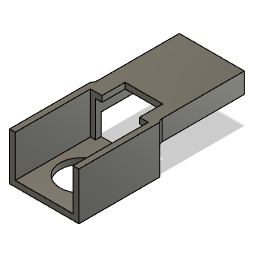
CMCz v3 (Autodesk Fusion 360 archive; units mm, degrees)
design "wire holder PIP modif"
Autodesk Fusion 360 part; units mm, degrees
note: some values were not read from the file. Chosen so that the rebuilt part matches the saved one: which face or edge a step refers to. Set by a fixed rule: which sketch regions a step uses.
sketch "Esquisse1" plane through (0, 0, 0) normal (0, 1, 0) x (1, 0, 0)
  line L0 (4.125, 6.5) -> (-4.125, 6.5)
  line L1 (-4.125, 6.5) -> (-4.125, -6.5)
  line L2 (-4.125, -6.5) -> (4.125, -6.5)
  line L3 (4.125, -6.5) -> (4.125, 6.5)
  line L4 (4.125, 6.5) -> (-4.125, -6.5) construction
  line L5 (-4.125, 6.5) -> (4.125, -6.5) construction
  line L6 (-5.625, -8) -> (5.625, -8)
  line L7 (5.625, -8) -> (5.625, 8)
  line L8 (5.625, 8) -> (-5.625, 8)
  line L9 (-5.625, 8) -> (-5.625, -8)
  line L10 (-1.375, 6.5) -> (-1.375, 8) construction
  line L11 (1.375, 6.5) -> (1.375, 8) construction
  line L12 (-1.875, 8) -> (-1.875, 6.5)
  line L13 (-0.875, 8) -> (-0.875, 6.5)
  line L14 (0.875, 8) -> (0.875, 6.5)
  line L15 (1.875, 8) -> (1.875, 6.5)
  line L16 (3.625, 8) -> (3.625, 6.5)
  line L17 (-3.625, 8) -> (-3.625, 6.5)
  line L18 (-4.125, -6.5) -> (-4.125, -8)
  line L19 (4.125, -6.5) -> (4.125, -4.6231)
  line L20 (4.125, -4.6231) -> (4.125, -8)
  dimension "d1" = 13
  dimension "d2" = 8.25
  dimension "d3" = 1.5
  dimension "d4" = 2.75
  dimension "d5" = 2.75
  dimension "d6" = 0.5
  dimension "d7" = 0.5
  dimension "d8" = 0.5
  dimension "d9" = 0.5
  dimension "d10" = 0.5
  dimension "d11" = 0.5
  dimension "d91" = 1.5
  constraint horizontal L0
  constraint perpendicular L0 L1
  constraint parallel L0 L2
  constraint parallel L1 L3
  constraint coincident L4 origin
  constraint coincident L5 origin
  constraint coincident L0 L10.start
  constraint coincident L8 L10.end
  constraint perpendicular L8 L10
  constraint coincident L0 L11.start
  constraint coincident L8 L11.end
  constraint perpendicular L8 L11
  constraint coincident L8 L12.start
  constraint coincident L0 L12.end
  constraint perpendicular L0 L12
  constraint coincident L8 L13.start
  constraint coincident L0 L13.end
  constraint perpendicular L0 L13
  constraint coincident L8 L14.start
  constraint coincident L0 L14.end
  constraint perpendicular L0 L14
  constraint coincident L8 L15.start
  constraint coincident L0 L15.end
  constraint perpendicular L0 L15
  constraint coincident L8 L16.start
  constraint coincident L0 L16.end
  constraint perpendicular L0 L16
  constraint coincident L8 L17.start
  constraint coincident L0 L17.end
  constraint perpendicular L0 L17
  constraint coincident L6 L18.end
  constraint perpendicular L6 L18
  constraint perpendicular L2 L19
  constraint coincident L6 L20.end
  constraint perpendicular L6 L20
  measures "d1" distance of L0.start L2.end
  measures "d2" distance of L0.start L0.end
  measures "d4" distance of L0.end L10.start
  measures "d5" distance of L10 L11
  measures "d6" horizontal distance of L0.end L17.start
  measures "d7" distance of L10 L12
  measures "d8" distance of L10 L13
  measures "d9" distance of L11 L14
  measures "d10" distance of L11 L15
  measures "d11" distance of L0.start L16
  measures "d91" distance of L1.end L18.end
extrude "Extrusion1" add sketch "Esquisse1" along normal blind 1
extrude "Extrusion2" add sketch "Esquisse1" against normal blind 2.5 contours L0 L3 L6 L7 L8 L16 L19 L20 | L0 L8 L14 L15 | L0 L1 L6 L8 L9 L17 L18 | L0 L8 L12 L13
sketch "Esquisse5" plane through (0, 1, 0) normal (0, 1, 0) x (-1, 0, 0)
  line L0 (5.625, -8) -> (5.625, 8)
  line L1 (5.625, 8) -> (-5.625, 8)
  line L2 (-5.625, 8) -> (-5.625, -8)
  line L3 (-5.625, -8) -> (5.625, -8)
  line L4 (5.625, 8) -> (-5.625, 8)
  line L5 (5, 8) -> (-5, 8)
  line L6 (-5, 8) -> (-5, 20)
  line L7 (-5, 20) -> (5, 20)
  line L8 (5, 20) -> (5, 8)
  line L9 (5.625, 8) -> (5.625, -8)
  line L10 (-5.625, -8) -> (-5.625, 8)
  line L11 (-6, 7) -> (-6, 21)
  line L12 (-6, 21) -> (6, 21)
  line L13 (6, 21) -> (6, 7)
  line L14 (6, 7) -> (-6, 7)
  line L15 (4.125, -6.5) -> (4.125, 8)
  line L16 (-4.125, 8) -> (-4.125, -6.5)
  point P0 (-4.125, 8)
  point P1 (0, 8)
  point P2 (0, 8)
  dimension "d33" = 10
  dimension "d34" = 12
  dimension "d35" = -1
  constraint horizontal L5
  constraint vertical L6
  constraint horizontal L7
  constraint vertical L8
  constraint coincident L5 P0
  constraint midpoint L4 P2
  constraint midpoint L5 P2
  constraint coincident P2 P1
  measures "d33" distance of L5.start L5.end
  measures "d34" distance of L5.end L6.end
extrude "Extrusion6" add sketch "Esquisse5" against normal blind 7.2 contours L0 L1 L4 L5 L9 L14 L15 | L0 L1 L2 L4 L6 L7 L8 L9 L10 L11 L12 L13 L14 | L1 L2 L4 L5 L10 L14 L16
sketch "Esquisse6" plane through (0, -6.2, 0) normal (0, -1, 0) x (1, 0, 0)
  line L0 (5, 20) -> (5, 8)
  line L1 (5, 8) -> (4.125, 8)
  line L2 (4.125, 8) -> (4.125, 7)
  line L3 (4.125, 7) -> (6, 7)
  line L4 (6, 7) -> (6, 21)
  line L5 (6, 21) -> (-6, 21)
  line L6 (-6, 21) -> (-6, 7)
  line L7 (-6, 7) -> (-4.125, 7)
  line L8 (-4.125, 7) -> (-4.125, 8)
  line L9 (-4.125, 8) -> (-5, 8)
  line L10 (-5, 8) -> (-5, 20)
  line L11 (-5, 20) -> (5, 20)
  line L12 (-6, 21) -> (6, 21)
  line L13 (6, 21) -> (6, 7)
  line L14 (6, 7) -> (-6, 7)
  line L15 (-6, 7) -> (-6, 21)
  circle A0 centre (0, 14.5) radius 3.75
  line L16 (0, 7) -> (0, 21) construction
  line L17 (-4.125, 8) -> (4.125, 8)
  dimension "d39" = 6.5
  dimension "d40" = 7.5
  constraint horizontal L12
  constraint vertical L13
  constraint horizontal L14
  constraint vertical L15
  constraint coincident L3.end L4.start
  constraint coincident L5.end L6.start
  constraint midpoint L14 L16.start
  constraint midpoint L5 L16.end
  constraint coincident A0.centre L16
  measures "d39" distance of A0.centre L17
  measures "d40" diameter of A0
extrude "Extrusion7" add sketch "Esquisse6" along normal blind 1
sketch "Esquisse9" plane through (0, 1, 0) normal (0, 1, 0) x (-1, 0, 0)
  line L0 (5, 8) -> (-5, 8)
  line L1 (-5, 8) -> (-5, 20)
  line L2 (-5, 20) -> (5, 20)
  line L3 (5, 20) -> (5, 8)
  line L4 (5.625, 7) -> (6, 7)
  line L5 (6, 7) -> (6, 21)
  line L6 (6, 21) -> (-6, 21)
  line L7 (-6, 21) -> (-6, 7)
  line L8 (-6, 7) -> (-5.625, 7)
  line L9 (-5.625, 7) -> (-5.625, -8)
  line L10 (-5.625, -8) -> (5.625, -8)
  line L11 (5.625, -8) -> (5.625, 7)
  line L12 (3, 8) -> (-3.5, 8)
  line L13 (-3.5, 8) -> (-3.5, 4)
  line L14 (-3.5, 4) -> (3, 4)
  line L15 (3, 4) -> (3, 8)
  dimension "d63" = 4
  dimension "d64" = 6.5
  dimension "d65" = 1.5
  constraint horizontal L12
  constraint vertical L13
  constraint horizontal L14
  constraint vertical L15
  constraint coincident L0 L12.start
  measures "d63" distance of L12.end L13.end
  measures "d64" distance of L13.end L14.end
  measures "d65" distance of L1 L12.end
extrude "Extrusion10" cut sketch "Esquisse9" against normal blind 2 contours L0 L12 L13 L14 L15
sketch "Esquisse10" plane through (0, 0, 7) normal (0, 0, -1) x (-1, 0, 0)
  line L0 (5.625, 1) -> (5.625, -2.5)
  line L1 (5.625, -2.5) -> (4.125, -2.5)
  line L2 (4.125, -2.5) -> (4.125, -6.2)
  line L3 (4.125, -6.2) -> (-4.125, -6.2)
  line L4 (-4.125, -6.2) -> (-4.125, -2.5)
  line L5 (-4.125, -2.5) -> (-5.625, -2.5)
  line L6 (-5.625, -2.5) -> (-5.625, 1)
  line L7 (-5.625, 1) -> (-6, 1)
  line L8 (-6, 1) -> (-6, -7.2)
  line L9 (-6, -7.2) -> (6, -7.2)
  line L10 (6, -7.2) -> (6, 1)
  line L11 (6, 1) -> (5.625, 1)
  line L12 (-6, -7.2) -> (6, -7.2)
  line L13 (6, -7.2) -> (6, -6.2)
  line L14 (6, -6.2) -> (-6, -6.2)
  line L15 (-6, -6.2) -> (-6, -7.2)
  line L16 (-5.625, -6.2) -> (-5.625, -7.2)
  line L17 (5.625, -6.2) -> (5.625, -7.2)
  constraint horizontal L12
  constraint vertical L13
  constraint horizontal L14
  constraint vertical L15
  constraint coincident L10 L13.end
  constraint coincident L8.end L9.start
  constraint collinear L3 L14
  constraint coincident L14 L16.start
  constraint coincident L12 L16.end
  constraint perpendicular L12 L16
  constraint coincident L14 L17.start
  constraint coincident L12 L17.end
  constraint perpendicular L12 L17
  constraint collinear L6 L16
  constraint collinear L0 L17
sketch "Esquisse11" plane through (0, -7.2, 0) normal (0, -1, 0) x (1, 0, 0)
  circle A0 centre (0, 14.5) radius 3.75
  line L0 (6, 7) -> (6, 21)
  line L1 (6, 21) -> (-6, 21)
  line L2 (-6, 21) -> (-6, 7)
  circle A1 centre (0, 4.5) radius 2.5
  line L3 (-6, 7) -> (6, 7)
  dimension "d72" = 10
  dimension "d73" = 5
  measures "d72" distance of A0.centre A1.centre
  measures "d73" diameter of A1
sketch "Esquisse12" plane through (0, -6.2, 0) normal (0, 1, 0) x (-1, 0, 0)
  line L0 (4.125, 7) -> (4.125, 8)
  line L1 (4.125, 8) -> (5, 8)
  line L2 (5, 8) -> (5, 20)
  line L3 (5, 20) -> (-5, 20)
  line L4 (-5, 20) -> (-5, 8)
  line L5 (-5, 8) -> (-4.125, 8)
  line L6 (-4.125, 8) -> (-4.125, 7)
  line L7 (-4.125, 7) -> (4.125, 7)
  circle A0 centre (0, 14.5) radius 3.75
  line L8 (4.125, 2.1) -> (4.125, 6)
  arc A1 (0.025, -2) -> (4.125, 2.1) centre (0.025, 2.1) ccw
  line L9 (-0.025, -2) -> (0.025, -2)
  arc A2 (-4.125, 2.1) -> (-0.025, -2) centre (-0.025, 2.1) ccw
  line L10 (-4.125, 6) -> (-4.125, 2.1)
  line L11 (-3.125, 6) -> (-4.125, 6)
  line L12 (-3.125, 9) -> (-3.125, 6)
  line L13 (-4, 9) -> (-3.125, 9)
  line L14 (-4, 19) -> (-4, 9)
  line L15 (4, 19) -> (-4, 19)
  line L16 (4, 9) -> (4, 19)
  line L17 (3.125, 9) -> (4, 9)
  line L18 (3.125, 6) -> (3.125, 9)
  line L19 (4.125, 6) -> (3.125, 6)
  line L20 (4.125, 7) -> (4.125, 6)
  line L21 (-4.125, 7) -> (-4.125, 6)
  line L22 (5.125, 1.85) -> (-5.125, 1.85)
  constraint coincident L0.start L7.end
  constraint coincident L6.end L7.start
  constraint parallel L7 L11
  constraint parallel L6 L12
  constraint parallel L5 L13
  constraint parallel L4 L14
  constraint parallel L3 L15
  constraint parallel L2 L16
  constraint parallel L1 L17
  constraint parallel L0 L18
  constraint tangent L8 A1
  constraint tangent A1 L9
  constraint tangent L9 A2
  constraint tangent A2 L10
sketch "Esquisse13" plane through (0, -7.2, 0) normal (0, -1, 0) x (1, 0, 0)
  line L0 (6, 7) -> (6, 21)
  line L1 (6, 21) -> (-6, 21)
  line L2 (-6, 21) -> (-6, 7)
  circle A0 centre (0, 14.5) radius 3.75
  circle A1 centre (0, 4.25) radius 3.5
  line L3 (-6, 7) -> (6, 7)
  dimension "d84" = 7
  measures "d84" diameter of A1
extrude "Extrusion15" cut 1 faces at (1.6667, -1.4, 20) along direction (0, 0, 1) blind 6
fillet "Congé3" radius 1 2 edges at (-5.625, -0.75, 7) (5.625, -0.75, 7)

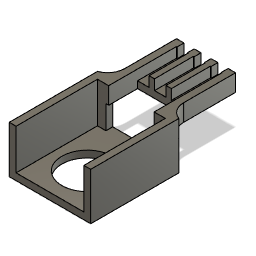
design "wire holder PIP midif v3"
Autodesk Fusion 360 part; units mm, degrees
sketch "Esquisse1" plane through (0, 0, 0) normal (0, 1, 0) x (1, 0, 0)
  line L0 (3.75, 4.5) -> (-3.75, 4.5)
  line L1 (-3.75, 4.5) -> (-3.75, -4.5)
  line L2 (-3.75, -4.5) -> (3.75, -4.5)
  line L3 (3.75, -4.5) -> (3.75, 4.5)
  line L4 (3.75, 4.5) -> (-3.75, -4.5) construction
  line L5 (-3.75, 4.5) -> (3.75, -4.5) construction
  line L6 (-4.75, -5.5) -> (4.75, -5.5)
  line L7 (4.75, -5.5) -> (4.75, 5.5)
  line L8 (4.75, 5.5) -> (-4.75, 5.5)
  line L9 (-4.75, 5.5) -> (-4.75, -5.5)
  line L10 (-1.25, 4.5) -> (-1.25, 5.5) construction
  line L11 (1.25, 4.5) -> (1.25, 5.5) construction
  line L12 (-1.75, 5.5) -> (-1.75, 4.5)
  line L13 (-0.75, 5.5) -> (-0.75, 4.5)
  line L14 (0.75, 5.5) -> (0.75, 4.5)
  line L15 (1.75, 5.5) -> (1.75, 4.5)
  line L16 (3.25, 5.5) -> (3.25, 4.5)
  line L17 (-3.25, 5.5) -> (-3.25, 4.5)
  line L18 (-3.75, -4.5) -> (-3.75, -5.5)
  line L19 (3.75, -4.5) -> (3.75, 15.3518)
  line L20 (3.75, 15.3518) -> (3.75, -5.5)
  line L21 (-1.65, 4.5) -> (-0.85, 4.5)
  line L22 (-0.85, 4.5) -> (-0.85, -5.5)
  line L23 (-0.85, -5.5) -> (-1.65, -5.5)
  line L24 (-1.65, -5.5) -> (-1.65, 4.5)
  line L25 (0.85, 4.5) -> (1.65, 4.5)
  line L26 (1.65, 4.5) -> (1.65, -5.5)
  line L27 (1.65, -5.5) -> (0.85, -5.5)
  line L28 (0.85, -5.5) -> (0.85, 4.5)
  line L29 (-3.35, 4.5) -> (-3.75, 4.5)
  line L30 (-3.75, 4.5) -> (-3.75, -5.5)
  line L31 (-3.75, -5.5) -> (-3.35, -5.5)
  line L32 (-3.35, -5.5) -> (-3.35, 4.5)
  line L33 (3.35, 4.5) -> (3.75, 4.5)
  line L34 (3.75, 4.5) -> (3.75, -5.5)
  line L35 (3.75, -5.5) -> (3.35, -5.5)
  line L36 (3.35, -5.5) -> (3.35, 4.5)
  line L37 (3.35, -5.5) -> (4.35, -5.5)
  line L38 (4.35, -5.5) -> (4.35, 5.5)
  line L39 (4.35, 5.5) -> (3.35, 5.5)
  line L40 (3.35, 5.5) -> (3.35, -5.5)
  line L41 (-3.35, -5.5) -> (-4.35, -5.5)
  line L42 (-4.35, -5.5) -> (-4.35, 5.5)
  line L43 (-4.35, 5.5) -> (-3.35, 5.5)
  line L44 (-3.35, 5.5) -> (-3.35, -5.5)
  dimension "d1" = 9
  dimension "d2" = 7.5
  dimension "d3" = 1
  dimension "d6" = 0.5
  dimension "d7" = 0.5
  dimension "d8" = 0.5
  dimension "d9" = 0.5
  dimension "d10" = 0.5
  dimension "d11" = 0.5
  dimension "d101" = 0.1
  dimension "d102" = 0.1
  dimension "d103" = 0.1
  dimension "d104" = 0.1
  dimension "d106" = 0.4
  dimension "d107" = 0.4
  dimension "d108" = 1.7
  dimension "d111" = 2.5
  dimension "d112" = 2.5
  dimension "d113" = 2.5
  dimension "d114" = 1.7
  dimension "d115" = 1.7
  dimension "d116" = 1
  dimension "d117" = 1
  constraint horizontal L0
  constraint perpendicular L0 L1
  constraint parallel L0 L2
  constraint parallel L1 L3
  constraint coincident L4 origin
  constraint coincident L5 origin
  constraint coincident L0 L10.start
  constraint coincident L8 L10.end
  constraint perpendicular L8 L10
  constraint coincident L0 L11.start
  constraint coincident L8 L11.end
  constraint perpendicular L8 L11
  constraint coincident L8 L12.start
  constraint coincident L0 L12.end
  constraint perpendicular L0 L12
  constraint coincident L8 L13.start
  constraint coincident L0 L13.end
  constraint perpendicular L0 L13
  constraint coincident L8 L14.start
  constraint coincident L0 L14.end
  constraint perpendicular L0 L14
  constraint coincident L8 L15.start
  constraint coincident L0 L15.end
  constraint perpendicular L0 L15
  constraint coincident L8 L16.start
  constraint coincident L0 L16.end
  constraint perpendicular L0 L16
  constraint coincident L8 L17.start
  constraint coincident L0 L17.end
  constraint perpendicular L0 L17
  constraint coincident L6 L18.end
  constraint perpendicular L6 L18
  constraint perpendicular L2 L19
  constraint coincident L6 L20.end
  constraint perpendicular L6 L20
  constraint horizontal L21
  constraint vertical L22
  constraint horizontal L23
  constraint vertical L24
  constraint coincident L0 L21.start
  constraint collinear L6 L23
  constraint horizontal L25
  constraint vertical L26
  constraint horizontal L27
  constraint vertical L28
  constraint coincident L6 L26.end
  constraint coincident L0 L25.start
  constraint horizontal L29
  constraint vertical L30
  constraint horizontal L31
  constraint vertical L32
  constraint coincident L0 L29.start
  constraint horizontal L33
  constraint vertical L34
  constraint horizontal L35
  constraint vertical L36
  constraint coincident L0 L33.start
  constraint horizontal L37
  constraint vertical L38
  constraint horizontal L39
  constraint vertical L40
  constraint coincident L8 L38.end
  constraint horizontal L41
  constraint vertical L42
  constraint horizontal L43
  constraint vertical L44
  constraint coincident L8 L42.end
  measures "d1" distance of L0.start L2.end
  measures "d2" distance of L0.start L0.end
  measures "d6" horizontal distance of L0.end L17.start
  measures "d7" distance of L10 L12
  measures "d8" distance of L10 L13
  measures "d9" distance of L11 L14
  measures "d10" distance of L11 L15
  measures "d11" distance of L0.start L16
  measures "d101" distance of L12 L24
  measures "d102" distance of L13 L22
  measures "d103" distance of L14 L28
  measures "d104" distance of L15 L26
  measures "d106" distance of L30 L32
  measures "d107" distance of L3 L36
  measures "d108" distance of L26 L36
  measures "d111" distance of L10 L30
  measures "d112" distance of L10 L11
  measures "d113" distance of L11 L34
  measures "d114" distance of L24 L32
  measures "d115" distance of L22 L28
  measures "d116" distance of L32 L42
  measures "d117" distance of L36 L38
extrude "Extrusion1" add sketch "Esquisse1" along normal blind 1 contours L0 L2 L3 L19 L20 L33 L34 L36 L40 | L3 L6 L8 L19 L20 L34 L37 L38 L39 | L0 L8 L19 L20 L33 L39 L40 | L0 L2 L26 L36 L40 | L0 L8 L16 L40 | L2 L6 L20 L34 L35 L36 L37 L40 | L0 L8 L15 L16 | L2 L6 L26 L36 L40 | L0 L8 L14 L15 L25 | L2 L6 L26 L27 L28 | L0 L2 L25 L26 L28 | L2 L6 L22 L28 | L0 L2 L22 L28 | L0 L8 L13 L14 | L2 L6 L22 L23 L24 | L0 L2 L21 L22 L24 | L0 L8 L12 L13 L21 | L2 L6 L24 L32 L44 | L0 L2 L24 L32 L44 | L0 L8 L12 L17 | L2 L6 L18 L30 L31 L32 L41 L44 | L0 L1 L2 L29 L30 L32 L44 | L0 L8 L17 L44 | L0 L1 L6 L8 L18 L29 L30 L41 L42 L43 L44
extrude "Extrusion2" add sketch "Esquisse1" against normal blind 1.75 contours L0 L2 L3 L19 L20 L33 L34 L36 L40 | L3 L6 L8 L19 L20 L34 L37 L38 L39 | L0 L8 L19 L20 L33 L39 L40 | L0 L8 L16 L40 | L2 L6 L20 L34 L35 L36 L37 L40 | L0 L8 L14 L15 L25 | L2 L6 L26 L27 L28 | L0 L2 L25 L26 L28 | L2 L6 L22 L23 L24 | L0 L2 L21 L22 L24 | L0 L8 L12 L13 L21 | L2 L6 L18 L30 L31 L32 L41 L44 | L0 L1 L2 L29 L30 L32 L44 | L0 L8 L17 L44 | L0 L1 L6 L8 L18 L29 L30 L41 L42 L43 L44
sketch "Esquisse5" plane through (0, 1, 0) normal (0, 1, 0) x (-1, 0, 0)
  line L0 (4.35, 5.5) -> (-4.35, 5.5)
  line L1 (-4.35, -5.5) -> (4.35, -5.5)
  line L2 (4.35, 5.5) -> (-4.35, 5.5)
  line L3 (5, 5.5) -> (-5, 5.5)
  line L4 (-5, 5.5) -> (-5, 17.5)
  line L5 (-5, 17.5) -> (5, 17.5)
  line L6 (5, 17.5) -> (5, 5.5)
  line L7 (4.75, 6.5) -> (4.75, -6.5)
  line L8 (-4.75, -6.5) -> (-4.75, 6.5)
  line L9 (-6, 4.5) -> (-6, 18.5)
  line L10 (-6, 18.5) -> (6, 18.5)
  line L11 (6, 18.5) -> (6, 4.5)
  line L12 (6, 4.5) -> (-6, 4.5)
  line L13 (3.75, -5.5) -> (3.75, 6.5)
  line L14 (-3.75, 6.5) -> (-3.75, -5.5)
  line L15 (-4.35, 5.5) -> (-4.35, -5.5)
  line L16 (4.35, -5.5) -> (4.35, 5.5)
  point P0 (0, 5.5)
  point P1 (0, 5.5)
  point P2 (-1.65, 5.5)
  point P3 (1.65, 5.5)
  point P4 (-3.35, 5.5)
  point P5 (-0.85, 5.5)
  point P6 (3.35, 5.5)
  point P7 (0.85, 5.5)
  dimension "d33" = 10
  dimension "d34" = 12
  dimension "d35" = -1
  constraint horizontal L3
  constraint vertical L4
  constraint horizontal L5
  constraint vertical L6
  constraint midpoint L2 P1
  constraint midpoint L3 P1
  constraint coincident P1 P0
  measures "d33" distance of L3.start L3.end
  measures "d34" distance of L3.end L4.end
extrude "Extrusion6" add sketch "Esquisse5" against normal blind 7.2 contours L0 L2 L3 L12 L13 L16 | L3 L7 L12 L16 | L3 L4 L5 L6 L7 L8 L9 L10 L11 L12 | L0 L2 L3 L12 L14 L15 | L3 L8 L12 L15
sketch "Esquisse6" plane through (0, -6.2, 0) normal (0, -1, 0) x (1, 0, 0)
  line L0 (5, 17.5) -> (5, 5.5)
  line L1 (5, 5.5) -> (3.75, 5.5)
  line L2 (3.75, 5.5) -> (3.75, 4.5)
  line L3 (3.75, 4.5) -> (6, 4.5)
  line L4 (6, 4.5) -> (6, 18.5)
  line L5 (6, 18.5) -> (-6, 18.5)
  line L6 (-6, 18.5) -> (-6, 4.5)
  line L7 (-6, 4.5) -> (-3.75, 4.5)
  line L8 (-3.75, 4.5) -> (-3.75, 5.5)
  line L9 (-3.75, 5.5) -> (-5, 5.5)
  line L10 (-5, 5.5) -> (-5, 17.5)
  line L11 (-5, 17.5) -> (5, 17.5)
  line L12 (-6, 18.5) -> (6, 18.5)
  line L13 (6, 18.5) -> (6, 4.5)
  line L14 (6, 4.5) -> (-6, 4.5)
  line L15 (-6, 4.5) -> (-6, 18.5)
  circle A0 centre (0, 12) radius 3.75
  line L16 (0, 4.5) -> (0, 18.5) construction
  line L17 (-3.35, 5.5) -> (-1.65, 5.5)
  line L18 (1.65, 5.5) -> (3.35, 5.5)
  line L19 (-0.85, 5.5) -> (0.85, 5.5)
  dimension "d40" = 7.5
  dimension "d133" = 6.5
  constraint horizontal L12
  constraint vertical L13
  constraint horizontal L14
  constraint vertical L15
  constraint coincident L3.end L4.start
  constraint coincident L5.end L6.start
  constraint midpoint L14 L16.start
  constraint midpoint L5 L16.end
  constraint coincident A0.centre L16
  measures "d40" diameter of A0
  measures "d133" distance of A0.centre L19
extrude "Extrusion7" add sketch "Esquisse6" along normal blind 1
sketch "Esquisse9" plane through (0, 1, 0) normal (0, 1, 0) x (-1, 0, 0)
  line L0 (-5, 5.5) -> (-5, 17.5)
  line L1 (-5, 17.5) -> (5, 17.5)
  line L2 (5, 17.5) -> (5, 5.5)
  line L3 (6, 4.5) -> (6, 18.5)
  line L4 (6, 18.5) -> (-6, 18.5)
  line L5 (-6, 18.5) -> (-6, 4.5)
  line L6 (-4.35, -5.5) -> (4.35, -5.5)
  line L7 (-4.35, 4.5) -> (-4.35, -5.5)
  line L8 (4.35, -5.5) -> (4.35, 4.5)
  line L9 (3.35, 5.5) -> (3.35, -4.5)
  line L10 (3.35, -4.5) -> (3.25, -4.5)
  line L11 (3.25, -4.5) -> (3.25, -5.5)
  line L12 (3.25, -5.5) -> (1.75, -5.5)
  line L13 (1.75, -5.5) -> (1.75, -4.5)
  line L14 (1.75, -4.5) -> (1.65, -4.5)
  line L15 (1.65, -4.5) -> (1.65, 5.5)
  line L16 (1.65, 5.5) -> (3.35, 5.5)
  line L17 (0.85, 5.5) -> (0.85, -4.5)
  line L18 (0.85, -4.5) -> (0.75, -4.5)
  line L19 (0.75, -4.5) -> (0.75, -5.5)
  line L20 (0.75, -5.5) -> (-0.75, -5.5)
  line L21 (-0.75, -5.5) -> (-0.75, -4.5)
  line L22 (-0.75, -4.5) -> (-0.85, -4.5)
  line L23 (-0.85, -4.5) -> (-0.85, 5.5)
  line L24 (-0.85, 5.5) -> (0.85, 5.5)
  line L25 (-3.25, -5.5) -> (-3.25, -4.5)
  line L26 (-3.25, -4.5) -> (-3.35, -4.5)
  line L27 (-3.35, -4.5) -> (-3.35, 5.5)
  line L28 (-3.35, 5.5) -> (-1.65, 5.5)
  line L29 (-1.65, 5.5) -> (-1.65, -4.5)
  line L30 (-1.65, -4.5) -> (-1.75, -4.5)
  line L31 (-1.75, -4.5) -> (-1.75, -5.5)
  line L32 (-1.75, -5.5) -> (-3.25, -5.5)
  line L33 (3.35, 5.5) -> (-3.35, 5.5)
  line L34 (-3.35, 5.5) -> (-3.35, 1.25)
  line L35 (-3.35, 1.25) -> (3.35, 1.25)
  line L36 (3.35, 1.25) -> (3.35, 5.5)
  dimension "d122" = 4.25
  constraint horizontal L33
  constraint vertical L34
  constraint horizontal L35
  constraint vertical L36
  constraint coincident L27 L34.end
  constraint coincident L9.start L16.end
  measures "d122" distance of L27.end L34.end
extrude "Extrusion10" cut sketch "Esquisse9" against normal blind 3.5 contours L27 L28 L29 L33 L34 L35 | L23 L29 L33 L35 | L17 L23 L24 L33 L35 | L15 L17 L33 L35 | L9 L15 L16 L33 L35 L36
sketch "Esquisse16" plane through (0, 0, 0) normal (0, -1, 0) x (1, 0, 0)
  line L0 (-1.65, 1.25) -> (-3.35, 1.25)
  line L1 (-3.35, 1.25) -> (-3.35, -4.5)
  line L2 (-3.35, -4.5) -> (-3.25, -4.5)
  line L3 (-3.25, -4.5) -> (-3.25, -5.5)
  line L4 (-3.25, -5.5) -> (-1.75, -5.5)
  line L5 (-1.75, -5.5) -> (-1.75, -4.5)
  line L6 (-1.75, -4.5) -> (-1.65, -4.5)
  line L7 (-1.65, -4.5) -> (-1.65, 1.25)
  line L8 (0.85, 1.25) -> (-0.85, 1.25)
  line L9 (-0.85, 1.25) -> (-0.85, -4.5)
  line L10 (-0.85, -4.5) -> (-0.75, -4.5)
  line L11 (-0.75, -4.5) -> (-0.75, -5.5)
  line L12 (-0.75, -5.5) -> (0.75, -5.5)
  line L13 (0.75, -5.5) -> (0.75, -4.5)
  line L14 (0.75, -4.5) -> (0.85, -4.5)
  line L15 (0.85, -4.5) -> (0.85, 1.25)
  line L16 (3.35, 1.25) -> (1.65, 1.25)
  line L17 (1.65, 1.25) -> (1.65, -4.5)
  line L18 (1.65, -4.5) -> (1.75, -4.5)
  line L19 (1.75, -4.5) -> (1.75, -5.5)
  line L20 (1.75, -5.5) -> (3.25, -5.5)
  line L21 (3.25, -5.5) -> (3.25, -4.5)
  line L22 (3.25, -4.5) -> (3.35, -4.5)
  line L23 (3.35, -4.5) -> (3.35, 1.25)
  line L24 (-3.35, 1.25) -> (3.35, 1.25)
  line L25 (3.35, 1.25) -> (3.35, -0.75)
  line L26 (3.35, -0.75) -> (-3.35, -0.75)
  line L27 (-3.35, -0.75) -> (-3.35, 1.25)
  dimension "d123" = 2
  constraint horizontal L24
  constraint vertical L25
  constraint horizontal L26
  constraint vertical L27
  constraint coincident L23 L25.end
  constraint coincident L0.end L1.start
  measures "d123" distance of L24 L26
extrude "Extrusion15" cut 1 faces at (1.6667, -1.4, 17.5) along direction (0, 0, 1) blind 6
sketch "Esquisse15" plane through (0, -7.2, 0) normal (0, -1, 0) x (1, 0, 0)
  circle A0 centre (0, 12) radius 3.75
  line L0 (6, 4.5) -> (6, 18.5)
  line L1 (6, 18.5) -> (-6, 18.5)
  line L2 (-6, 18.5) -> (-6, 4.5)
  line L3 (-6, 18.5) -> (6, 18.5)
  line L4 (6, 18.5) -> (6, 17.5)
  line L5 (6, 17.5) -> (-6, 17.5)
  line L6 (-6, 17.5) -> (-6, 18.5)
  line L7 (-6, 4.5) -> (6, 4.5)
  dimension "d98" = 1
  constraint horizontal L3
  constraint vertical L4
  constraint horizontal L5
  constraint vertical L6
  constraint coincident L0 L4.end
  constraint coincident L1.end L2.start
  measures "d98" distance of L3 L5
extrude "Extrusion17" cut sketch "Esquisse15" against normal blind 16 contours L0 L1 L2 L3 L4 L5 L6
fillet "Congé3" radius 2.5 2 edges at (-4.35, -0.375, 4.5) (4.35, -0.375, 4.5)
ref_plane "Plan de construction1" through (4.625, -2.25, 0) normal (0, -1, 0) x (0, 0, -1)
sketch "Esquisse18" plane through (4.625, -2.25, 0) normal (0, -1, 0) x (1, 0, 0)
  line L0 (-8.375, 4.5) -> (-10.625, 4.5)
  arc A0 (-8.975, 2.1489) -> (-10.625, 4.5) centre (-11.475, 2.1489) ccw
  line L1 (-8.975, 2.1489) -> (-8.975, -5.5)
  line L2 (-8.975, -5.5) -> (-7.875, -5.5)
  line L3 (-7.875, -5.5) -> (-7.875, -4.5)
  line L4 (-7.875, -4.5) -> (-7.975, -4.5)
  line L5 (-7.975, -4.5) -> (-7.975, 5.5)
  line L6 (-7.975, 5.5) -> (-8.375, 5.5)
  line L7 (-8.375, 5.5) -> (-8.375, 4.5)
  line L8 (-5.475, 1.25) -> (-6.275, 1.25)
  line L9 (-6.275, 1.25) -> (-6.275, -4.5)
  line L10 (-6.275, -4.5) -> (-6.375, -4.5)
  line L11 (-6.375, -4.5) -> (-6.375, -5.5)
  line L12 (-6.375, -5.5) -> (-5.375, -5.5)
  line L13 (-5.375, -5.5) -> (-5.375, -4.5)
  line L14 (-5.375, -4.5) -> (-5.475, -4.5)
  line L15 (-5.475, -4.5) -> (-5.475, 1.25)
  line L16 (-2.975, 1.25) -> (-3.775, 1.25)
  line L17 (-3.775, 1.25) -> (-3.775, -4.5)
  line L18 (-3.775, -4.5) -> (-3.875, -4.5)
  line L19 (-3.875, -4.5) -> (-3.875, -5.5)
  line L20 (-3.875, -5.5) -> (-2.875, -5.5)
  line L21 (-2.875, -5.5) -> (-2.875, -4.5)
  line L22 (-2.875, -4.5) -> (-2.975, -4.5)
  line L23 (-2.975, -4.5) -> (-2.975, 1.25)
  line L24 (-0.875, 4.5) -> (-0.875, 5.5)
  line L25 (-0.875, 5.5) -> (-1.275, 5.5)
  line L26 (-1.275, 5.5) -> (-1.275, -4.5)
  line L27 (-1.275, -4.5) -> (-1.375, -4.5)
  line L28 (-1.375, -4.5) -> (-1.375, -5.5)
  line L29 (-1.375, -5.5) -> (-0.275, -5.5)
  line L30 (-0.275, -5.5) -> (-0.275, 2.1489)
  arc A1 (1.375, 4.5) -> (-0.275, 2.1489) centre (2.225, 2.1489) ccw
  line L31 (1.375, 4.5) -> (-0.875, 4.5)
  line L32 (-6.275, 0.05) -> (-6.275, 1.25)
  line L33 (-6.275, 1.25) -> (-7.975, 1.25)
  line L34 (-7.975, 1.25) -> (-7.975, 0.05)
  line L35 (-7.975, 0.05) -> (-6.275, 0.05)
  line L36 (-3.775, 0.05) -> (-3.775, 1.25)
  line L37 (-3.775, 1.25) -> (-5.475, 1.25)
  line L38 (-5.475, 1.25) -> (-5.475, 0.05)
  line L39 (-5.475, 0.05) -> (-3.775, 0.05)
  line L40 (-2.975, 1.25) -> (-2.975, 0.05)
  line L41 (-2.975, 0.05) -> (-1.275, 0.05)
  line L42 (-1.275, 0.05) -> (-1.275, 1.25)
  line L43 (-1.275, 1.25) -> (-2.975, 1.25)
  line L44 (-2.975, 1.25) -> (-2.975, -4.5)
  line L45 (-2.975, -4.5) -> (-2.875, -4.5)
  line L46 (-2.875, -4.5) -> (-2.875, -5.5)
  line L47 (-2.875, -5.5) -> (-1.375, -5.5)
  line L48 (-1.375, -5.5) -> (-1.375, -4.5)
  line L49 (-1.375, -4.5) -> (-1.275, -4.5)
  line L50 (-1.275, -4.5) -> (-1.275, 1.25)
  line L51 (-5.475, 1.25) -> (-5.475, -4.5)
  line L52 (-5.475, -4.5) -> (-5.375, -4.5)
  line L53 (-5.375, -4.5) -> (-5.375, -5.5)
  line L54 (-5.375, -5.5) -> (-3.875, -5.5)
  line L55 (-3.875, -5.5) -> (-3.875, -4.5)
  line L56 (-3.875, -4.5) -> (-3.775, -4.5)
  line L57 (-3.775, -4.5) -> (-3.775, 1.25)
  line L58 (-7.975, -4.5) -> (-7.975, 5.5)
  line L59 (-7.975, 1.25) -> (-7.975, -4.5)
  line L60 (-7.975, -4.5) -> (-7.875, -4.5)
  line L61 (-7.875, -4.5) -> (-7.875, -5.5)
  line L62 (-7.875, -5.5) -> (-6.375, -5.5)
  line L63 (-6.375, -5.5) -> (-6.375, -4.5)
  line L64 (-6.375, -4.5) -> (-6.275, -4.5)
  line L65 (-6.275, -4.5) -> (-6.275, 1.25)
  line L66 (-1.275, 1.25) -> (-2.975, 1.25)
  line L67 (-3.775, 1.25) -> (-5.475, 1.25)
  line L68 (-6.275, 1.25) -> (-7.975, 1.25)
sketch "Esquisse19" plane through (0, 0, -5.5) normal (0, 0, -1) x (-1, 0, 0)
  line L0 (-3.25, 0) -> (-1.75, 0)
  line L1 (-1.75, 0) -> (-1.75, -1.75)
  line L2 (-1.75, -1.75) -> (-0.75, -1.75)
  line L3 (-0.75, -1.75) -> (-0.75, 0)
  line L4 (-0.75, 0) -> (0.75, 0)
  line L5 (0.75, 0) -> (0.75, -1.75)
  line L6 (0.75, -1.75) -> (1.75, -1.75)
  line L7 (1.75, -1.75) -> (1.75, 0)
  line L8 (1.75, 0) -> (3.25, 0)
  line L9 (3.25, 0) -> (3.25, -1.75)
  line L10 (3.25, -1.75) -> (4.35, -1.75)
  line L11 (4.35, -1.75) -> (4.35, 1)
  line L12 (4.35, 1) -> (-4.35, 1)
  line L13 (-4.35, 1) -> (-4.35, -1.75)
  line L14 (-4.35, -1.75) -> (-3.25, -1.75)
  line L15 (-3.25, -1.75) -> (-3.25, 0)
  line L16 (-6, -1.75) -> (-4.35, -1.75)
  line L17 (-4.35, -1.75) -> (-4.35, 1)
  line L18 (-6, 1) -> (-4.35, 1)
  line L19 (-6, 1) -> (-6, -1.75)
  line L20 (4.35, -1.75) -> (4.35, 1)
  line L21 (6, 1) -> (4.35, 1)
  line L22 (4.35, 1) -> (4.35, -1.75)
  line L23 (6, -1.75) -> (4.35, -1.75)
  line L24 (6, -1.75) -> (6, 1)
  line L25 (-6, -1.75) -> (6, -1.75)
  line L26 (6, -1.75) -> (6, 1)
  line L27 (6, 1) -> (-6, 1)
  line L28 (-6, 1) -> (-6, -1.75)
  constraint horizontal L25
  constraint vertical L26
  constraint horizontal L27
  constraint vertical L28
  constraint coincident L21.start L24.end
  constraint coincident L16.start L19.end
extrude "Extrusion20" cut sketch "Esquisse19" against normal up to surface (10 mm away) contours L0 L1 L2 L3 L4 L5 L6 L7 L8 L9 L10 L11 L12 L13 L14 L15 L17 L20 L22 L25 L27 | L13 L16 L17 L18 L19 L25 L27 L28 | L11 L20 L21 L22 L23 L24 L25 L26 L27
extrude "Extrusion21" add sketch "Esquisse18" along normal blind 1
extrude "Extrusion22" cut sketch "Esquisse18" against normal blind 7 contours L0 A0 L1 L2 L3 L4 L5 L6 L7 L34 L58 L59 L60 L61 | L8 L9 L10 L11 L12 L13 L14 L15 L32 L38 L51 L52 L53 L63 L64 L65 | L16 L17 L18 L19 L20 L21 L22 L23 L36 L40 L44 L45 L46 L55 L56 L57 | L24 L25 L26 L27 L28 L29 L30 A1 L31 L42 L48 L49 L50
extrude "Extrusion23" add sketch "Esquisse18" against normal blind 2 contours L0 A0 L1 L2 L3 L4 L5 L6 L7 L34 L58 L59 L60 L61 | L8 L9 L10 L11 L12 L13 L14 L15 L32 L38 L51 L52 L53 L63 L64 L65 | L16 L17 L18 L19 L20 L21 L22 L23 L36 L40 L44 L45 L46 L55 L56 L57 | L24 L25 L26 L27 L28 L29 L30 A1 L31 L42 L48 L49 L50
extrude "Extrusion24" cut 1 faces at (1.1167, -3.25, -3.25) along direction (0, 1, 0) blind 0.5
extrude "Extrusion25" add 3 faces at (2.25, -2.25, -0.6667) (-0.25, -2.25, -0.6667) (-2.75, -2.25, -0.6667) along direction (0, 1, 0) blind 0.5
extrude "Extrusion26" cut 2 faces at (-5.6667, 1, 9.1667) (5.6667, 1, 9.1667) along direction (0, 1, 0) up to surface end surface through (4.625, -0.25, 0) normal (0, 1, 0) offset 0

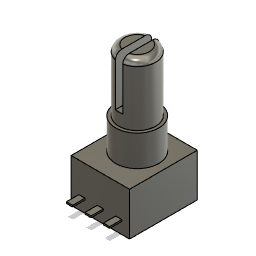
design "poto"
Autodesk Fusion 360 part; units mm, degrees
sketch "Esquisse1" plane through (0, 0, 0) normal (0, 1, 0) x (1, 0, 0)
  line L0 (4.75, 5.5) -> (-4.75, 5.5)
  line L1 (-4.75, 5.5) -> (-4.75, -5.5)
  line L2 (-4.75, -5.5) -> (4.75, -5.5)
  line L3 (4.75, -5.5) -> (4.75, 5.5)
  line L4 (4.75, 5.5) -> (-4.75, -5.5) construction
  line L5 (-4.75, 5.5) -> (4.75, -5.5) construction
  dimension "d1" = 11
  dimension "d2" = 9.5
  constraint horizontal L0
  constraint perpendicular L0 L1
  constraint parallel L0 L2
  constraint parallel L1 L3
  constraint coincident L4 origin
  constraint coincident L5 origin
  measures "d1" distance of L0.start L2.end
  measures "d2" distance of L0.start L0.end
extrude "Extrusion1" add sketch "Esquisse1" along normal blind 7
sketch "Esquisse2" plane through (0, 7, 0) normal (0, 1, 0) x (-1, 0, 0)
  line L0 (-4.75, 5.5) -> (-4.75, -5.5)
  line L1 (-4.75, -5.5) -> (4.75, -5.5)
  line L2 (4.75, -5.5) -> (4.75, 5.5)
  line L3 (4.75, 5.5) -> (-4.75, 5.5)
  circle A0 centre (0, -0.5) radius 3.5
  dimension "d5" = 7
  dimension "d27" = 5
  measures "d5" diameter of A0
  measures "d27" distance of L1 A0.centre
extrude "Extrusion2" add sketch "Esquisse2" along normal blind 5 contours A0
sketch "Esquisse3" plane through (0, 12, 0) normal (0, 1, 0) x (-1, 0, 0)
  circle A0 centre (0, -0.5) radius 3.5
  circle A1 centre (0, -0.5) radius 3
  dimension "d8" = 6
  constraint concentric A0 A1
  measures "d8" diameter of A1
extrude "Extrusion3" add sketch "Esquisse3" along normal blind 10 contours A1
sketch "Esquisse4" plane through (0, 22, 0) normal (0, 1, 0) x (-1, 0, 0)
  circle A0 centre (0, -0.5) radius 3
  circle A1 centre (0, -0.5) radius 3
  line L0 (0.6, -3.4394) -> (0.6, 2.4394)
  line L1 (-0.6, -3.4394) -> (-0.6, 2.4394)
  dimension "d11" = 0.6
  dimension "d12" = 0.6
  constraint coincident A1 L0.start
  constraint coincident A1 L0.end
  constraint vertical L0
  constraint coincident A1 L1.start
  constraint coincident A1 L1.end
  constraint parallel L0 L1
  measures "d11" horizontal distance of origin L0.start
  measures "d12" horizontal distance of origin L1.start
extrude "Extrusion4" cut sketch "Esquisse4" against normal blind 8 contours A0 A1 L0 L1
fillet "Congé1" radius 1 3 edges at (-2.3238, 22, -2.3974) (3, 22, -0.5) (-2.3238, 22, 1.3974)
sketch "Esquisse5" plane through (0, 0, 5.5) normal (0, 0, 1) x (1, 0, 0)
  line L0 (-4.75, 0) -> (4.75, 0)
  line L1 (4.75, 0) -> (4.75, 7)
  line L2 (4.75, 7) -> (-4.75, 7)
  line L3 (-4.75, 7) -> (-4.75, 0)
  line L4 (0.5041, 2.125) -> (-0.4959, 2.125)
  line L5 (-0.4959, 2.125) -> (-0.4959, 1.875)
  line L6 (-0.4959, 1.875) -> (0.5041, 1.875)
  line L7 (0.5041, 1.875) -> (0.5041, 2.125)
  line L8 (0.5041, 2.125) -> (-0.4959, 1.875) construction
  line L9 (-0.4959, 2.125) -> (0.5041, 1.875) construction
  line L10 (0, 0) -> (0, 7) construction
  line L11 (-3.4959, 1.875) -> (-2.4959, 1.875)
  line L12 (-3.4959, 2.125) -> (-3.4959, 1.875)
  line L13 (-2.4959, 2.125) -> (-3.4959, 2.125)
  line L14 (-2.4959, 2.125) -> (-3.4959, 1.875) construction
  line L15 (-2.4959, 1.875) -> (-2.4959, 2.125)
  line L16 (-3.4959, 2.125) -> (-2.4959, 1.875) construction
  line L17 (2.5041, 1.875) -> (3.5041, 1.875)
  line L18 (2.5041, 2.125) -> (2.5041, 1.875)
  line L19 (3.5041, 2.125) -> (2.5041, 2.125)
  line L20 (3.5041, 2.125) -> (2.5041, 1.875) construction
  line L21 (3.5041, 1.875) -> (3.5041, 2.125)
  line L22 (2.5041, 2.125) -> (3.5041, 1.875) construction
  point P0 (0.0041, 2)
  dimension "d18" = 1
  dimension "d19" = 0.25
  dimension "d20" = 2
  dimension "d23" = 3
  dimension "d24" = 0
  constraint horizontal L4
  constraint perpendicular L4 L5
  constraint parallel L4 L6
  constraint parallel L5 L7
  constraint coincident L8 P0
  constraint coincident L9 P0
  constraint coincident L10.start origin
  constraint midpoint L2 L10.end
  measures "d18" distance of L4.start L4.end
  measures "d19" distance of L4.start L6.end
  measures "d20" vertical distance of L10.start P0
extrude "Extrusion5" add sketch "Esquisse5" along normal blind 2 contours L4 L5 L6 L7 | L11 L12 L13 L15 | L17 L18 L19 L21
